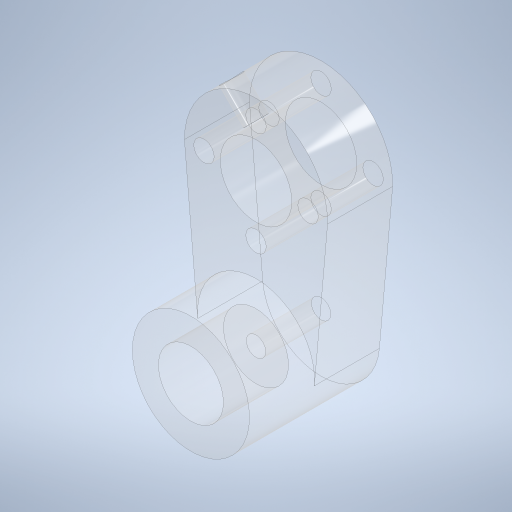
# Autodesk Inventor part: кривошип
Saved by Autodesk Inventor 2023.1 (Build 271208000, 208)
## iProperties
Created: 2024-12-17
Part Number: кривошип
Material: Пластик САН
Document SubType Name: Modeling
Designer: DELL
Density: 1.068 g/cm^3
Appearance: Поликарбонат — прозрачный
Mass: 8.5101 g
Surface Area: 40.8775 cm^2
Volume: 7.96826 cm^3
Author: DELL
Autodesk Inventor part; units mm, degrees
ref_plane "YZ Plane" through (0, 0, 0) normal (1, 0, 0) x (0, 1, 0)
sketch "Эскиз1" plane through (0, 0, 0) normal (0, 0, 1) x (1, 0, 0)
  circle A0 centre (-1.7368, -21.67) radius 2.375 projected
  circle A1 centre (-1.7368, -21.67) radius 7.5
  line L0 (-1.7368, -14.17) -> (-1.7368, -54.17) construction
  arc A2 (5.7632, -21.67) -> (-9.2368, -21.67) centre (-1.7368, -21.67) ccw
  circle A3 centre (-1.7368, -43.67) radius 9
  circle A4 centre (-1.7368, -43.67) radius 1.5
  circle A5 centre (-1.7368, -43.67) radius 5
  line L1 (-10.7368, -43.67) -> (-9.2368, -21.67)
  line L2 (7.2632, -43.67) -> (5.7632, -21.67)
  point P0 (0, 0)
  point P1 (-1.7368, -34.17)
  dimension "d1" = 15
  dimension "d3" = 18
  dimension "d4" = 3
  dimension "d9" = 10
  dimension "d36" = 22
  constraints: 8 end point, 5 point on circle, 4 centre point, 3 coincident, 2 point on line, 1 midpoint, 1 vertical, 1 vertical alignment, 2 other
  measures "d3" diameter of A3
  measures "d4" diameter of A4
  measures "d9" diameter of A5
  measures "d36" distance of A0.centre A3.centre
extrude "Выдавливание1" add sketch "Эскиз1" along normal blind 20 contours L2 A3 L1 | A3 L2 | L1 A3
ref_plane "РабПлоскость1" through (0, 0, 0) normal (0, 0, 1) x (1, 0, 0)
sketch "Эскиз2" plane through (0, 0, 0) normal (0, 0, 1) x (1, 0, 0)
  arc A0 (-10.7011, -44.4704) -> (7.2269, -44.4779) centre (-1.7368, -43.67) ccw
  circle A1 centre (-1.7368, -46.2892) radius 1.5 construction
  line L0 (-1.7368, -46.2892) -> (-1.7368, -6.2497) construction
  line L1 (55.1846, -47.0725) -> (61.6072, -35.9345) construction
  line L2 (61.6072, -35.9345) -> (57.2758, -33.4368) construction
  line L3 (57.2758, -33.4368) -> (59.7378, -29.1672) construction
  line L4 (59.7378, -29.1672) -> (54.2369, -25.9951) construction
  line L5 (54.2369, -25.9951) -> (53.6124, -27.078) construction
  line L6 (53.6124, -27.078) -> (51.62, -25.929) construction
  line L7 (51.62, -25.929) -> (52.2444, -24.8462) construction
  line L8 (52.2444, -24.8462) -> (46.7434, -21.6741) construction
  line L9 (46.7434, -21.6741) -> (48.2421, -19.0752) construction
  line L10 (48.2421, -19.0752) -> (53.743, -22.2473) construction
  line L11 (53.743, -22.2473) -> (54.3674, -21.1644) construction
  line L12 (54.3674, -21.1644) -> (56.3599, -22.3134) construction
  line L13 (56.3599, -22.3134) -> (55.7355, -23.3962) construction
  line L14 (55.7355, -23.3962) -> (61.2364, -26.5683) construction
  line L15 (61.2364, -26.5683) -> (63.6984, -22.2987) construction
  line L16 (63.6984, -22.2987) -> (68.0299, -24.7964) construction
  line L17 (68.0299, -24.7964) -> (74.4526, -13.6584) construction
  line L18 (74.4526, -13.6584) -> (23.3414, 15.8145) construction
  arc A2 (23.3414, 15.8145) -> (19.2439, 14.7142) centre (21.8428, 13.2156) ccw construction
  line L19 (19.2439, 14.7142) -> (16.6854, 10.2772) construction
  arc A3 (12.8035, 9.064) -> (16.6854, 10.2772) centre (14.0865, 11.7758) ccw construction
  arc A4 (12.8035, 9.064) -> (-21.0534, -49.6498) centre (-1.7368, -21.67) ccw construction
  arc A5 (-20.1589, -53.6172) -> (-21.0534, -49.6498) centre (-22.7578, -52.1186) ccw construction
  line L20 (-20.1589, -53.6172) -> (-22.7175, -58.0542) construction
  arc A6 (-22.7175, -58.0542) -> (-21.6172, -62.1517) centre (-20.1186, -59.5528) ccw construction
  line L21 (-21.6172, -62.1517) -> (29.4939, -91.6246) construction
  line L22 (29.4939, -91.6246) -> (35.9166, -80.4866) construction
  line L23 (35.9166, -80.4866) -> (31.5851, -77.9889) construction
  line L24 (31.5851, -77.9889) -> (34.0472, -73.7193) construction
  line L25 (34.0472, -73.7193) -> (28.5462, -70.5472) construction
  line L26 (28.5462, -70.5472) -> (27.9218, -71.6301) construction
  line L27 (27.9218, -71.6301) -> (25.9293, -70.4811) construction
  line L28 (25.9293, -70.4811) -> (26.5537, -69.3983) construction
  line L29 (26.5537, -69.3983) -> (21.0528, -66.2262) construction
  line L30 (21.0528, -66.2262) -> (22.5514, -63.6273) construction
  line L31 (22.5514, -63.6273) -> (28.0524, -66.7994) construction
  line L32 (28.0524, -66.7994) -> (28.6768, -65.7165) construction
  line L33 (28.6768, -65.7165) -> (30.6693, -66.8655) construction
  line L34 (30.6693, -66.8655) -> (30.0448, -67.9483) construction
  line L35 (30.0448, -67.9483) -> (35.5458, -71.1204) construction
  line L36 (35.5458, -71.1204) -> (38.0078, -66.8508) construction
  line L37 (38.0078, -66.8508) -> (42.3393, -69.3485) construction
  line L38 (42.3393, -69.3485) -> (48.7619, -58.2105) construction
  line L39 (48.7619, -58.2105) -> (44.4305, -55.7128) construction
  line L40 (44.4305, -55.7128) -> (50.8531, -44.5748) construction
  line L41 (50.8531, -44.5748) -> (55.1846, -47.0725) construction
  circle A7 centre (-1.7368, -21.67) radius 2.375 construction
  circle A8 centre (-1.7368, -21.67) radius 5.5
  arc A9 (9.1272, -23.3947) -> (-12.5628, -23.6187) centre (-1.7368, -21.67) ccw
  line L42 (-12.7368, -21.67) -> (-10.7011, -44.4704)
  circle A10 centre (-1.7368, -43.67) radius 9 construction
  line L43 (9.2605, -21.9158) -> (7.2269, -44.4779)
  circle A11 centre (-1.7368, -43.67) radius 1.5
  circle A12 centre (-1.7368, -13.67) radius 1.575
  circle A13 centre (6.2632, -21.67) radius 1.575
  circle A14 centre (-1.7368, -29.67) radius 1.575
  circle A15 centre (-9.7368, -21.67) radius 1.575
  point P0 (0, 0)
  point P1 (-1.7368, -12.095)
  point P2 (-1.7368, -10.67)
  point P3 (-1.7368, -10.67)
  point P4 (7.8382, -21.67)
  point P5 (-1.7368, -31.245)
  point P6 (-11.3118, -21.67)
  dimension "d22" = 3.15
  dimension "d20" = 11
  dimension "d21" = 22
  dimension "d27" = 8
  dimension "d30" = 360
  constraints: 9 point on circle, 7 coincident, 6 end point, 5 centre point, 5 point on line, 2 horizontal alignment, 2 tangent, 2 vertical alignment, 1 equal radius, 1 vertical, 23 other
  measures "d20" diameter of A8
  measures "d21" diameter of A9
  measures "d27" distance of A4.centre point (-1.737, -13.67)
extrude "Выдавливание2" add sketch "Эскиз2" along normal blind 10 contours L42 A9 L43 A0
ref_plane "РабПлоскость5" through (-9.7368, -21.67, 0) normal (-0.7071068, 0.7071068, 0) x (0, 0, 1)
sketch "Эскиз4" plane through (-9.7368, -21.67, 0) normal (-0.7071068, 0.7071068, 0) x (0, 0, 1)
  line L0 (10, 1.575) -> (0, 1.575) construction
  line L1 (0, 9.7387) -> (10, 9.7387) construction
  line L2 (10, -3.8949) -> (0, -3.8949) construction
  line L3 (0, -3.8949) -> (0, -1.575) construction
  line L4 (0, -1.575) -> (10, -1.575) construction
  line L5 (10, -1.575) -> (10, -3.8949) construction
  line L6 (0, 15.0908) -> (10, 15.0908) construction
  line L7 (10, 15.0908) -> (10, 12.8887) construction
  line L8 (10, 12.8887) -> (0, 12.8887) construction
  line L9 (0, 12.8887) -> (0, 15.0908) construction
  line L10 (10, 1.575) -> (10, -1.575) construction
  line L11 (0, 12.8887) -> (0, 9.7387) construction
  circle A0 centre (6, 5.6568) radius 1.575
  line L12 (0, 1.575) -> (0, 9.7387) projected
  line L13 (10, 9.7387) -> (10, 1.575) projected
  point P0 (0, 22.208)
  dimension "d32" = 3.15
  constraints: 1 centre point
  measures "d32" diameter of A0
extrude "Выдавливание4" cut sketch "Эскиз4" along normal blind 10
